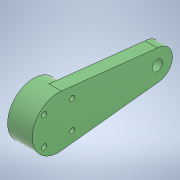
# Autodesk Inventor part: Biellette moteur-doigts
Saved by Autodesk Inventor 2022 (Build 260153000, 153)
## iProperties
Created: 2022-01-07
Part Number: Biellette moteur-doigts
Material: Générique
Document SubType Name: Modeling
Designer: victo
Density: 1 g/cm^3
Appearance: Lisse - Vert forêt foncé
Author: victo
Autodesk Inventor part; units mm, degrees
ref_plane "YZ Plane" through (0, 0, 0) normal (1, 0, 0) x (0, 1, 0)
ref_plane "XZ Plane" through (0, 0, 0) normal (0, 1, 0) x (-1, 0, 0)
ref_plane "XY Plane" through (0, 0, 0) normal (0, 0, 1) x (1, 0, 0)
sketch "Esquisse2" plane through (0, 0, 0) normal (-1, 0, 0) x (0, 0, 1)
  circle A0 centre (0, 0) radius 8 construction
  circle A1 centre (0, 0) radius 10.5
  line L0 (0, 0) -> (5.6569, 5.6569) construction
  line L1 (0, 0) -> (8, 0) construction
  circle A2 centre (5.6569, 5.6569) radius 1.05
  circle A3 centre (-5.6569, 5.6569) radius 1.05
  circle A4 centre (-5.6569, -5.6569) radius 1.05
  circle A5 centre (5.6569, -5.6569) radius 1.05
  circle A6 centre (0, 0) radius 2 projected
  dimension "d30" = 16
  dimension "d13" = 45
  dimension "d14" = 2.1
  dimension "d17" = 360
  dimension "d29" = 21
  constraints: 6 coincident, 5 centre point, 4 end point, 1 equal length, 1 horizontal, 12 other
  measures "d13" angle of L1 L0
  measures "d14" diameter of A2
  measures "d29" diameter of A1
extrude "Extrusion5" add sketch "Esquisse2" along normal blind 5 contours A1 | A6
sketch "Esquisse6" plane through (0, 0, 0) normal (0, 1, 0) x (-1, 0, 0)
  circle A0 centre (7.5, 0) radius 3.5
  line L0 (4, 0) -> (7.5, 0)
  line L1 (10.8, 0) -> (-1.8, 0) projected
  line L2 (5, -10.5) -> (5, 10.5) projected
  point P0 (0, 0)
  point P1 (5, 0)
  point P2 (5, 2.4495)
  dimension "d46" = 7
  dimension "d48" = 1
  constraints: 2 end point, 1 horizontal, 1 point on line, 3 other
  measures "d48" distance from line of L2 L0.start
revolve "Révolution1" cut sketch "Esquisse6" angle 360 about axis through (-4, 0, 0) along (-1, 0, 0) picked at (4.8584, 1.4572) contours L2 L0 A0
sketch "Esquisse7" plane through (0, 0, 0) normal (1, 0, 0) x (0, 0, -1)
  circle A0 centre (0, 0) radius 10.5 projected
  circle A1 centre (-5.6569, -5.6569) radius 1.05 projected
  circle A2 centre (5.6569, -5.6569) radius 1.05 projected
  circle A3 centre (5.6569, 5.6569) radius 1.05 projected
  circle A4 centre (-5.6569, 5.6569) radius 1.05 projected
  circle A5 centre (0, 0) radius 10.5 projected
  line L0 (0, 10.5652) -> (40, 6.1)
  line L1 (40, 6.1) -> (40, -6.1)
  line L2 (40, -6.1) -> (0, -10.5652)
  line L3 (0, -10.5652) -> (0, 10.5652)
  arc A6 (40, -6.1) -> (40, 6.1) centre (40, 0) ccw
  circle A7 centre (40, 0) radius 2.1
  line L4 (0, -14.7913) -> (0, 14.7913) projected
  line L5 (57.42, 0) -> (-21.82, 0) projected
  point P0 (1.1649, 10.4352)
  point P1 (1.1649, -10.4352)
  dimension "d49" = 40
  dimension "d53" = 4.2
  dimension "d54" = 4
  constraints: 8 end point, 2 centre point, 2 point on circle, 2 tangent, 1 coincident, 1 collinear, 1 midpoint, 1 parallel, 1 point on line
  measures "d49" distance between parallel lines of L1 L3
  measures "d53" diameter of A7
  measures "d54" radial gap between concentric circles of A6 A7
extrude "Extrusion9" add sketch "Esquisse7" along normal blind 5 contours L5 L3 A0 | L5 A7 L1 L2 A0 | A0 L0 L1 A7 L5 | A0 L3 L5 | L5 A0 L3 | L3 A0 L5 | A6 L5 A7 L1 | L1 A7 L5 A6
